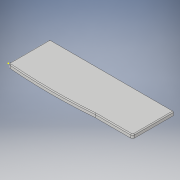
# Autodesk Inventor part: key board low tec
Saved by Autodesk Inventor 2017 (Build 210142000, 142)
## iProperties
Created: 2018-03-14
Part Number: key board low tec
Material: Generic
Document SubType Name: Modeling
Designer: braxtonwright
Density: 1 g/cm^3
Appearance: Default
Author: braxtonwright
Autodesk Inventor part; units mm, degrees
ref_plane "YZ Plane" through (0, 0, 0) normal (1, 0, 0) x (0, 1, 0)
ref_plane "XZ Plane" through (0, 0, 0) normal (0, 1, 0) x (-1, 0, 0)
ref_plane "XY Plane" through (0, 0, 0) normal (0, 0, 1) x (1, 0, 0)
sketch "Sketch1" plane through (0, 0, 0) normal (0, 1, 0) x (-1, 0, 0)
  line L0 (-25.9292, 0) -> (-36.5125, 0)
  line L1 (-37.0417, -0.5292) -> (-37.0417, -12.1708)
  line L2 (-37.0417, -12.1708) -> (0, -12.1708)
  line L3 (0, -12.1708) -> (0, -0.5292)
  arc A0 (0, -0.5292) -> (-0.5292, 0) centre (-0.5292, -0.5292) ccw
  line L4 (-18.5208, -12.969) -> (-18.5208, 2.8326) construction
  arc A1 (-36.5125, 0) -> (-37.0417, -0.5292) centre (-36.5125, -0.5292) ccw
  arc A2 (-0.5292, 0) -> (-25.9292, 0) centre (-13.2292, -152.1354) ccw
  point P0 (0, 0)
  point P1 (-13.2292, 0.5292)
  dimension "d4" = 1.0583
  dimension "d5" = 12.1708
  dimension "d6" = 37.0417
  dimension "d9" = 25.4
  dimension "d10" = 0.5292
  constraints: 10 end point, 7 point on circle, 3 centre point, 3 perpendicular, 1 horizontal, 1 symmetric about line, 1 vertical, 1 other
  measures "d4" diameter of A0
  measures "d5" distance between parallel lines of L0 L2
  measures "d6" distance between parallel lines of L1 L3
  measures "d9" distance of L0.start A0.end
  measures "d10" distance from line of L0 point (-13.229, 0.529)
extrude "main key board" add sketch "Sketch1" along normal blind 1.0583
fillet "Fillet1" radius 0.254 6 edges at (0.155, 1.0583, -0.155) (0, 1.0583, -6.35) (13.2292, 1.0583, 0.5292) (36.8867, 1.0583, -0.155) (37.0417, 1.0583, -6.35) (31.2208, 1.0583, 0)
sketch "Sketch2" plane through (0, 1.0583, 0) normal (0, 1, 0) x (1, 0, 0)
  point P0 (0, 0)
body "Solid1"
